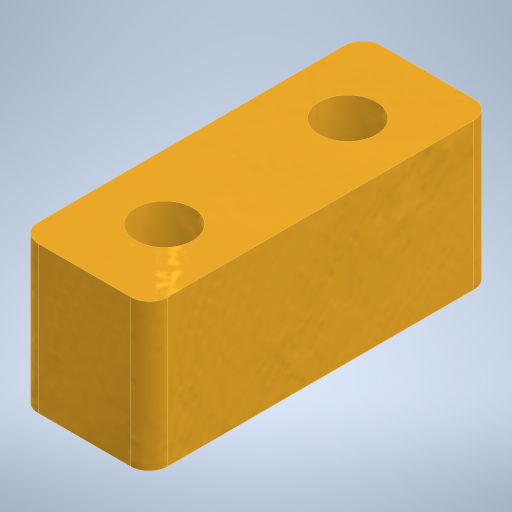
# Autodesk Inventor part: креп_сервы
Saved by Autodesk Inventor 2023.1 (Build 271208000, 208)
## iProperties
Created: 2025-02-07
Part Number: креп_сервы
Material: Типовые
Document SubType Name: Modeling
Designer: baranovaem
Density: 1 g/cm^3
Appearance: Сварка — латунь
Author: baranovaem
Autodesk Inventor part; units mm, degrees
ref_plane "YZ Plane" through (0, 0, 0) normal (1, 0, 0) x (0, 1, 0)
ref_plane "XZ Plane" through (0, 0, 0) normal (0, 1, 0) x (-1, 0, 0)
ref_plane "XY Plane" through (0, 0, 0) normal (0, 0, 1) x (1, 0, 0)
sketch "Эскиз1" plane through (0, 0, 0) normal (0, 1, 0) x (-1, 0, 0)
  circle A0 centre (0, -5) radius 1.55
  circle A1 centre (0, 5) radius 1.55
  line L0 (0, 5) -> (0, -5) construction
  line L1 (3.525, 9.35) -> (-3.525, 9.35)
  line L2 (-3.525, 9.35) -> (-3.525, -9.35)
  line L3 (-3.525, -9.35) -> (3.525, -9.35)
  line L4 (3.525, -9.35) -> (3.525, 9.35)
  line L5 (3.525, 9.35) -> (-3.525, -9.35) construction
  line L6 (-3.525, 9.35) -> (3.525, -9.35) construction
  point P0 (0, 0)
  point P1 (0, 0)
  dimension "d2" = 3.1
  dimension "d3" = 3.1
  dimension "d4" = 10
  dimension "d5" = 7.05
  dimension "d6" = 18.7
  constraints: 14 end point, 3 coincident, 3 midpoint, 2 centre point, 2 parallel, 1 horizontal, 1 perpendicular, 1 vertical
  measures "d2" diameter of A0
  measures "d3" diameter of A1
  measures "d4" distance of L0.start L0.end
  measures "d5" distance of L3.end L2.end
  measures "d6" distance of L2.end L1.end
extrude "Выдавливание1" add sketch "Эскиз1" along normal blind 8
fillet "Сопряжение1" radius 1 4 edges at (-3.525, 4, 9.35) (3.525, 4, 9.35) (3.525, 4, -9.35) (-3.525, 4, -9.35)
